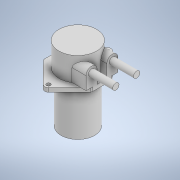
# Autodesk Inventor part: peristaltic pump
Saved by Autodesk Inventor 2022 (Build 260153000, 153)
## iProperties
Created: 2021-12-03
Part Number: peristaltic pump
Material: Generic
Document SubType Name: Modeling
Designer: efred
Density: 1 g/cm^3
Appearance: Default
Author: efred
Autodesk Inventor part; units mm, degrees
ref_plane "YZ Plane" through (0, 0, 0) normal (1, 0, 0) x (0, 1, 0)
ref_plane "XZ Plane" through (0, 0, 0) normal (0, 1, 0) x (-1, 0, 0)
ref_plane "XY Plane" through (0, 0, 0) normal (0, 0, 1) x (1, 0, 0)
sketch "Sketch1" plane through (0, 0, 0) normal (0, 1, 0) x (-1, 0, 0)
  circle A0 centre (0, 0) radius 13.8
  dimension "d0" = 27.6
  constraints: 1 centre point, 1 coincident
  measures "d0" diameter of A0
extrude "Extrusion1" add sketch "Sketch1" along normal blind 38.2
sketch "Sketch2" plane through (0, 38.2, 0) normal (0, 1, 0) x (1, 0, 0)
  line L0 (-19.85, -8.5) -> (19.85, -8.5) construction
  line L1 (19.85, -7.6776) -> (19.85, 7.6776)
  line L2 (19.85, 8.5) -> (-19.85, 8.5) construction
  line L3 (-19.85, 7.6776) -> (-19.85, -7.6776)
  line L4 (-19.2715, -9.0845) -> (-2.2034, -26.3306)
  line L5 (-2.2034, -26.3306) -> (2.2034, -26.3306) construction
  line L6 (2.2034, -26.3306) -> (19.2715, -9.0845)
  arc A0 (-2.2034, -26.3306) -> (2.2034, -26.3306) centre (0, -24.15) ccw
  circle A1 centre (0, -24.15) radius 1.6
  line L7 (-19.85, 0) -> (19.85, 0) construction
  line L8 (-19.2715, 9.0845) -> (-2.2034, 26.3306)
  line L9 (2.2034, 26.3306) -> (19.2715, 9.0845)
  arc A2 (2.2034, 26.3306) -> (-2.2034, 26.3306) centre (0, 24.15) ccw
  circle A3 centre (0, 24.15) radius 1.6
  arc A4 (-19.85, -7.6776) -> (-19.2715, -9.0845) centre (-17.85, -7.6776) ccw
  arc A5 (-19.2715, 9.0845) -> (-19.85, 7.6776) centre (-17.85, 7.6776) ccw
  arc A6 (19.85, 7.6776) -> (19.2715, 9.0845) centre (17.85, 7.6776) ccw
  arc A7 (19.2715, -9.0845) -> (19.85, -7.6776) centre (17.85, -7.6776) ccw
  point P0 (0, 0)
  point P1 (0, 8.5)
  point P2 (0, -27.25)
  dimension "d3" = 39.7
  dimension "d4" = 17
  dimension "d6" = 3.2
  dimension "d7" = 1.5
  dimension "d8" = 27.25
  dimension "d9" = 2
  constraints: 20 end point, 13 point on circle, 9 tangent, 8 centre point, 8 point on line, 4 symmetric about line, 3 equal radius, 3 midpoint, 3 vertical alignment, 2 coincident, 2 horizontal, 2 parallel, 1 horizontal alignment, 1 perpendicular, 2 other
  measures "d3" distance between parallel lines of L1 L3
  measures "d4" distance between parallel lines of L2 L0
  measures "d6" diameter of A1
  measures "d7" radial gap between concentric circles of A1 A0
  measures "d8" distance of point (0, 0) point (0, -27.25)
  measures "d9" radius of A4
extrude "Extrusion2" add sketch "Sketch2" along normal blind 3.3
sketch "Sketch3" plane through (0, 41.5, 0) normal (0, 1, 0) x (1, 0, 0)
  circle A0 centre (0, 0) radius 13.8 construction
  circle A1 centre (0, 0) radius 15.5
  dimension "d12" = 31
  constraints: 1 centre point, 1 coincident
  measures "d12" diameter of A1
extrude "Extrusion3" add sketch "Sketch3" along normal blind 19.5
sketch "Sketch4" plane through (19.85, 38.2, 7.6776) normal (1, 0, 0) x (0, 0, -1)
  line L0 (23.1776, 22.8) -> (-7.8224, 22.8) projected
  line L1 (-7.8224, 3.3) -> (23.1776, 3.3) construction
  line L2 (-7.8224, 3.3) -> (-7.8224, 22.8) projected
  line L3 (23.1776, 3.3) -> (23.1776, 22.8) projected
  line L4 (3.6776, 18.5) -> (11.6776, 18.5)
  line L5 (11.6776, 18.5) -> (11.6776, 3.3)
  line L6 (11.6776, 3.3) -> (3.6776, 3.3)
  line L7 (3.6776, 3.3) -> (3.6776, 18.5)
  line L8 (0, 3.3) -> (15.3553, 3.3) projected
  line L9 (3.6776, 18.5) -> (-5.4224, 18.5)
  line L10 (-5.4224, 18.5) -> (-5.4224, 3.3)
  line L11 (-5.4224, 3.3) -> (3.6776, 3.3)
  line L12 (3.6776, 3.3) -> (3.6776, 18.5)
  line L13 (7.6776, 3.3) -> (7.6776, 18.5) construction
  arc A0 (3.6776, 13.95) -> (-5.4224, 13.95) centre (-0.8724, 13.95) ccw
  line L14 (20.7776, 18.5) -> (20.7776, 3.3)
  line L15 (20.7776, 3.3) -> (11.6776, 3.3)
  arc A1 (20.7776, 13.95) -> (11.6776, 13.95) centre (16.2276, 13.95) ccw
  point P0 (7.6776, -38.2)
  point P1 (11.6776, 13.95)
  point P2 (3.6776, 13.95)
  dimension "d15" = 8
  dimension "d16" = 15.2
  dimension "d17" = 9.1
  constraints: 22 end point, 6 symmetric about line, 4 parallel, 4 point on circle, 4 point on line, 3 midpoint, 3 tangent, 2 centre point, 2 horizontal, 2 perpendicular, 1 coincident, 1 collinear, 1 other
  measures "d15" distance between parallel lines of L5 L7
  measures "d16" distance between parallel lines of L1 L4
  measures "d17" distance between parallel lines of L10 L7
extrude "Extrusion4" add sketch "Sketch4" against normal up to surface contours L7 L8 L11 L10 A0 | A1 L14 L15 L8 L5
sketch "Sketch5" plane through (19.85, 38.2, 7.6776) normal (1, 0, 0) x (0, 0, -1)
  arc A0 (3.6776, 13.95) -> (-5.4224, 13.95) centre (-0.8724, 13.95) ccw projected
  arc A1 (20.7776, 13.95) -> (11.6776, 13.95) centre (16.2276, 13.95) ccw projected
  circle A2 centre (-0.8724, 13.95) radius 2.6
  circle A3 centre (16.2276, 13.95) radius 2.6
  point P0 (7.6776, -38.2)
  dimension "d20" = 5.2
  dimension "d21" = 5.2
  constraints: 2 centre point, 2 coincident
  measures "d20" diameter of A2
  measures "d21" diameter of A3
extrude "Extrusion5" add sketch "Sketch5" along normal blind 20
equation "\"d18\" = d16"
body "Solid1"
